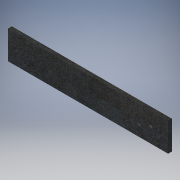
# Autodesk Inventor part: ballastBar
Saved by Autodesk Inventor 2016 (Build 200138000, 138)
## iProperties
Created: 2015-12-25
Part Number: ballastBar
Material: Steel
Document SubType Name: Modeling
Designer: Artur
Density: 7.85 g/cm^3
Appearance: Plate
Mass: 124.468 g
Surface Area: 97.467 cm^2
Volume: 15.8558 cm^3
Author: Artur
Autodesk Inventor part; units mm, degrees
ref_plane "YZ Plane" through (0, 0, 0) normal (1, 0, 0) x (0, 1, 0)
ref_plane "XZ Plane" through (0, 0, 0) normal (0, 1, 0) x (-1, 0, 0)
ref_plane "XY Plane" through (0, 0, 0) normal (0, 0, 1) x (1, 0, 0)
sketch "Sketch1" plane through (0, 0, 0) normal (0, 1, 0) x (-1, 0, 0)
  line L0 (0, 0) -> (169, 0)
  line L1 (169, 0) -> (169, -30)
  line L2 (169, -30) -> (0, -30)
  line L3 (0, -30) -> (0, 0)
  dimension "d0" = 169
  dimension "d1" = 30
  constraints: 8 end point, 2 parallel, 1 horizontal, 1 perpendicular
  measures "d0" distance of L0.start L0.end
  measures "d1" distance of L0.end L1.end
extrude "Extrusion1" add sketch "Sketch1" along normal blind 4
sketch "Sketch2" plane through (0, 0, 0) normal (0, -1, 0) x (1, 0, 0)
  line L0 (0, 0) -> (0, -30) projected
  line L1 (0, -15) -> (-169, -15) construction
  line L2 (-169, -30) -> (-169, 0) projected
  line L3 (-84.5, -15) -> (-84.5, 52.7002) construction
  point P0 (-161.5, -15)
  point P1 (-7.5, -15)
  dimension "d6" = 154
  constraints: 4 end point, 3 midpoint, 1 point on line, 1 symmetric about line, 1 vertical
  measures "d6" diameter of point (-161.5, -15) L3
hole "Hole1" at (-161.5, 0, -15) at (-7.5, 0, -15) direction (0, 1, 0) diameter 4 end through all
sketch "Sketch3" plane through (0, 0, 0) normal (0, -1, 0) x (1, 0, 0)
  line L0 (-169, -30) -> (-169, 0) construction
  line L1 (-169, -15) -> (0, -15) construction
  line L2 (0, 0) -> (0, -30) construction
  line L3 (-169, -4.25) -> (0, -4.25)
  line L4 (-169, -4.25) -> (-169, -15)
  line L5 (0, -4.25) -> (0, -15)
  line L6 (-169, -25.75) -> (0, -25.75)
  line L7 (-169, -25.75) -> (-169, -15)
  line L8 (0, -25.75) -> (0, -15)
  dimension "d15" = 21.5
  constraints: 14 end point, 2 collinear, 2 midpoint, 2 point on line, 2 symmetric about line, 1 perpendicular
  measures "d15" diameter of L3 L1
extrude "Extrusion2" [suppressed]
body "Solid1"
